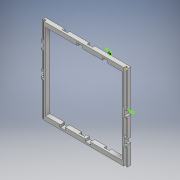
# Autodesk Inventor part: Female_Final
Saved by Autodesk Inventor 2017 (Build 210142000, 142)
## iProperties
Created: 2018-11-26
Part Number: Female_Final
Material: Generic
Document SubType Name: Modeling
Designer: Ralph
Density: 1 g/cm^3
Appearance: Default
Author: Ralph
Autodesk Inventor part; units mm, degrees
ref_plane "YZ Plane" through (0, 0, 0) normal (1, 0, 0) x (0, 1, 0)
ref_plane "XZ Plane" through (0, 0, 0) normal (0, 1, 0) x (-1, 0, 0)
ref_plane "XY Plane" through (0, 0, 0) normal (0, 0, 1) x (1, 0, 0)
sketch "Sketch1" plane through (0, 0, 0) normal (0, 1, 0) x (-1, 0, 0)
  line L0 (0, 0) -> (100, 0)
  line L1 (100, 0) -> (100, -100)
  line L2 (100, -100) -> (0, -100)
  line L3 (0, -100) -> (0, 0)
  line L4 (5, -5) -> (95, -5)
  line L5 (95, -5) -> (95, -95)
  line L6 (95, -95) -> (5, -95)
  line L7 (5, -95) -> (5, -5)
  line L8 (0, 0) -> (0, -5)
  line L9 (0, -5) -> (5, -5)
  dimension "d0" = 100
  dimension "d1" = 100
  dimension "d2" = 90
  dimension "d3" = 90
  dimension "d4" = 5
  dimension "d5" = 5
  constraints: 20 end point, 4 parallel, 3 perpendicular, 2 horizontal, 1 point on line
  measures "d0" distance of L1.end L2.end
  measures "d1" distance of L0.end L1.end
  measures "d2" distance of L5.end L6.end
  measures "d3" distance of L4.end L5.end
  measures "d4" distance between parallel lines of L0 L9
  measures "d5" distance between parallel lines of L3 L7
extrude "Extrusion1" add sketch "Sketch1" along normal blind 5
sketch "Sketch2" plane through (0, 0, 0) normal (0, -1, 0) x (1, 0, 0)
  circle A0 centre (-20, 6) radius 2
  line L0 (-20, 6) -> (-23.9485, 9.8906)
  line L1 (-23.9485, 9.8906) -> (-21.7943, 9.8906)
  line L2 (-21.7943, 9.8906) -> (-23.9485, 9.8906)
  line L3 (-23.9485, 9.8906) -> (-23.9485, 7.9453)
  arc A1 (2.0531, -40.1608) -> (5.7851, -40.1608) centre (3.9191, -39.7302) ccw
  arc A2 (9.4213, -40.1608) -> (5.7851, -40.1608) centre (7.6032, -41.1873) ccw
  point P0 (0, 0)
  dimension "d8" = 4
  constraints: 8 end point, 4 point on circle, 3 centre point, 1 collinear, 1 horizontal, 1 vertical
  measures "d8" diameter of A0
sketch "Sketch3" plane through (0, 0, 0) normal (0, -1, 0) x (1, 0, 0)
  line L0 (0, 0) -> (0, -100) projected
  line L1 (0, 0) -> (0, -5)
  line L2 (0, -5) -> (-20, -5)
  line L3 (-5, -5) -> (-95, -5) projected
  line L4 (-20, -5) -> (-30, -5)
  line L5 (-30, -5) -> (-50, -5)
  line L6 (-50, -5) -> (-60, -5)
  line L7 (-100, -100) -> (-100, 0) projected
  line L8 (-100, -100) -> (-100, -95)
  line L9 (-100, -95) -> (-80, -95)
  line L10 (-95, -95) -> (-5, -95) projected
  line L11 (-80, -95) -> (-70, -95)
  line L12 (-70, -95) -> (-50, -95)
  line L13 (-50, -95) -> (-40, -95)
  line L14 (-20, -5) -> (-22.75, -5)
  line L15 (-22.75, -5) -> (-28.25, -5)
  line L16 (-28.25, -5) -> (-28.25, -2.25)
  line L17 (-28.25, -2.25) -> (-22.75, -2.25)
  line L18 (-22.75, -2.25) -> (-22.75, -5)
  line L19 (-60, -5) -> (-57.25, -5)
  line L20 (-57.25, -5) -> (-51.75, -5)
  line L21 (-51.75, -5) -> (-51.75, -2.25)
  line L22 (-51.75, -2.25) -> (-57.25, -2.25)
  line L23 (-57.25, -2.25) -> (-57.25, -5)
  line L24 (-40, -95) -> (-42.75, -95)
  line L25 (-42.75, -95) -> (-48.25, -95)
  line L26 (-48.25, -95) -> (-48.25, -97.75)
  line L27 (-48.25, -97.75) -> (-42.75, -97.75)
  line L28 (-42.75, -97.75) -> (-42.75, -95)
  line L29 (-80, -95) -> (-77.25, -95)
  line L30 (-77.25, -95) -> (-71.75, -95)
  line L31 (-71.75, -95) -> (-71.75, -97.75)
  line L32 (-71.75, -97.75) -> (-77.25, -97.75)
  line L33 (-77.25, -97.75) -> (-77.25, -95)
  dimension "d9" = 5
  dimension "d10" = 20
  dimension "d11" = 10
  dimension "d12" = 20
  dimension "d13" = 10
  dimension "d14" = 5
  dimension "d15" = 20
  dimension "d16" = 10
  dimension "d17" = 20
  dimension "d18" = 10
  dimension "d19" = 2.75
  dimension "d20" = 5.5
  dimension "d21" = 2.75
  dimension "d22" = 2.75
  dimension "d23" = 5.5
  dimension "d24" = 2.75
  dimension "d25" = 2.75
  dimension "d26" = 5.5
  dimension "d27" = 2.75
  dimension "d28" = 2.75
  dimension "d29" = 5.5
  dimension "d30" = 2.75
  constraints: 60 end point, 13 point on line, 8 parallel, 4 horizontal, 4 perpendicular, 1 midpoint
  measures "d9" distance of L0.start L1.end
  measures "d10" distance of L1.end L2.end
  measures "d11" distance of L2.end L4.end
  measures "d12" distance of L4.end L5.end
  measures "d13" distance of L5.end L6.end
  measures "d14" distance of L7.start L8.end
  measures "d15" distance of L8.end L9.end
  measures "d16" distance of L9.end L11.end
  measures "d17" distance of L11.end L12.end
  measures "d18" distance of L12.end L13.end
  measures "d19" distance of L2.end L14.end
  measures "d20" distance of L16.end L17.end
  measures "d21" distance of L15.end L16.end
  measures "d22" distance of L6.end L19.end
  measures "d23" distance of L22.end L21.end
  measures "d24" distance of L21.end L20.end
  measures "d25" distance of L13.end L24.end
  measures "d26" distance of L27.end L26.end
  measures "d27" distance of L26.end L25.end
  measures "d28" distance of L9.end L29.end
  measures "d29" distance of L31.end L32.end
  measures "d30" distance of L30.end L31.end
extrude "Extrusion2" cut sketch "Sketch3" against normal blind 3
sketch "Sketch4" plane through (0, 0, 0) normal (0, -1, 0) x (1, 0, 0)
  line L0 (0, 0) -> (-3.25, 0)
  line L1 (-3.25, 0) -> (-3.25, -100)
  line L2 (-3.25, -100) -> (0, -100)
  line L3 (0, -100) -> (0, 0)
  line L4 (-100, 0) -> (0, 0) projected
  line L5 (-100, 0) -> (-96.75, 0)
  line L6 (-96.75, 0) -> (-96.75, -100)
  line L7 (-96.75, -100) -> (-100, -100)
  line L8 (-100, -100) -> (-100, 0)
  dimension "d33" = 3.25
  dimension "d34" = 100
  dimension "d35" = 3.25
  dimension "d36" = 100
  constraints: 16 end point, 4 parallel, 2 horizontal, 2 perpendicular
  measures "d33" distance of L2.end L1.end
  measures "d34" distance of L1.end L0.end
  measures "d35" distance of L6.end L7.end
  measures "d36" distance of L5.end L6.end
extrude "Extrusion3" cut sketch "Sketch4" against normal blind 1
sketch "Sketch5" plane through (0, 1, 0) normal (0, -1, 0) x (1, 0, 0)
  line L0 (-3.25, -100) -> (-3.25, 0) projected
  line L1 (-3.25, 0) -> (-1.25, 0)
  line L2 (-1.25, 0) -> (-1.25, -100)
  line L3 (-1.25, -100) -> (-3.25, -100)
  line L4 (-3.25, -100) -> (-3.25, 0)
  line L5 (-96.75, 0) -> (-3.25, 0) projected
  line L6 (-96.75, 0) -> (-98.75, 0)
  line L7 (-98.75, 0) -> (-98.75, -100)
  line L8 (-98.75, -100) -> (-96.75, -100)
  line L9 (-96.75, -100) -> (-96.75, 0)
  point P0 (0, 0)
  dimension "d39" = 2
  dimension "d40" = 100
  dimension "d41" = 2
  dimension "d42" = 100
  constraints: 16 end point, 4 parallel, 2 horizontal, 2 perpendicular
  measures "d39" distance of L2.end L3.end
  measures "d40" distance of L1.end L2.end
  measures "d41" distance of L8.end L7.end
  measures "d42" distance of L7.end L6.end
extrude "Extrusion4" cut sketch "Sketch5" against normal blind 1.75
sketch "Sketch6" plane through (-5, 5, -5) normal (0, 0, -1) x (-1, 0, 0)
  line L0 (17.75, -2) -> (23.25, -2) projected
  line L1 (23.25, -2) -> (17.25, -2)
  line L2 (17.25, -2) -> (17.25, 0)
  line L3 (17.25, 0) -> (23.25, 0)
  line L4 (23.25, 0) -> (23.25, -2)
  line L5 (46.75, -5) -> (46.75, -2) projected
  line L6 (46.75, -2) -> (52.75, -2)
  line L7 (52.75, -2) -> (52.75, 0)
  line L8 (52.75, 0) -> (46.75, 0)
  line L9 (46.75, 0) -> (46.75, -2)
  point P0 (-5, -5)
  dimension "d47" = 6
  dimension "d48" = 2
  dimension "d49" = 6
  dimension "d50" = 2
  constraints: 16 end point, 4 parallel, 2 horizontal, 2 perpendicular
  measures "d47" distance of L2.end L3.end
  measures "d48" distance of L1.end L2.end
  measures "d49" distance of L8.end L7.end
  measures "d50" distance of L7.end L6.end
extrude "Extrusion5" cut sketch "Sketch6" against normal blind 2.75
sketch "Sketch7" plane through (-95, 5, -95) normal (0, 0, 1) x (1, 0, 0)
  line L0 (17.75, -2) -> (23.25, -2) projected
  line L1 (23.25, -2) -> (17.25, -2)
  line L2 (17.25, -2) -> (17.25, 0)
  line L3 (17.25, 0) -> (23.25, 0)
  line L4 (23.25, 0) -> (23.25, -2)
  line L5 (46.75, -5) -> (46.75, -2) projected
  line L6 (46.75, -2) -> (52.75, -2)
  line L7 (52.75, -2) -> (52.75, 0)
  line L8 (52.75, 0) -> (46.75, 0)
  line L9 (46.75, 0) -> (46.75, -2)
  point P0 (95, -5)
  dimension "d53" = 6
  dimension "d54" = 2
  dimension "d55" = 6
  dimension "d56" = 2
  constraints: 16 end point, 4 parallel, 2 horizontal, 2 perpendicular
  measures "d53" distance of L2.end L3.end
  measures "d54" distance of L1.end L2.end
  measures "d55" distance of L8.end L7.end
  measures "d56" distance of L7.end L6.end
extrude "Extrusion6" cut sketch "Sketch7" against normal blind 2.75
fillet "Fillet1" radius 1 4 edges at (-77.25, 0, -96.375) (-42.75, 0, -96.375) (-22.75, 0, -3.625) (-57.25, 0, -3.625)
sketch "Sketch8" plane through (-100, 5, 0) normal (0, 0, 1) x (1, 0, 0)
  line L0 (0, -4) -> (0, 0) projected
  line L1 (0, 0) -> (20, 0)
  line L2 (20, 0) -> (30, 0)
  line L3 (30, 0) -> (50, 0)
  line L4 (50, 0) -> (60, 0)
  line L5 (60, 0) -> (57, 0)
  line L6 (0, 0) -> (100, 0) projected
  line L7 (57, 0) -> (51.5, 0)
  line L8 (51.5, 0) -> (51.5, -2.75)
  line L9 (51.5, -2.75) -> (57, -2.75)
  line L10 (57, -2.75) -> (57, 0)
  line L11 (20, 0) -> (23, 0)
  line L12 (23, 0) -> (28.5, 0)
  line L13 (28.5, 0) -> (28.5, -2.75)
  line L14 (28.5, -2.75) -> (23, -2.75)
  line L15 (23, -2.75) -> (23, 0)
  point P0 (100, -5)
  dimension "d60" = 20
  dimension "d61" = 10
  dimension "d62" = 20
  dimension "d63" = 10
  dimension "d64" = 3
  dimension "d65" = 5.5
  dimension "d66" = 2.75
  dimension "d67" = 3
  dimension "d68" = 5.5
  dimension "d69" = 2.75
  constraints: 28 end point, 5 point on line, 4 parallel, 3 horizontal, 2 perpendicular
  measures "d60" distance of L0.end L1.end
  measures "d61" distance of L1.end L2.end
  measures "d62" distance of L2.end L3.end
  measures "d63" distance of L3.end L4.end
  measures "d64" distance of L4.end L5.end
  measures "d65" distance of L9.end L8.end
  measures "d66" distance of L8.end L7.end
  measures "d67" distance of L1.end L11.end
  measures "d68" distance of L13.end L14.end
  measures "d69" distance of L12.end L13.end
extrude "Extrusion7" cut sketch "Sketch8" against normal blind 3
sketch "Sketch9" plane through (0, 5, 0) normal (0, 1, 0) x (1, 0, 0)
  line L0 (-43, 3) -> (-48.5, 3) projected
  line L1 (-48.5, 3) -> (-42.5, 3)
  line L2 (-42.5, 3) -> (-42.5, 5)
  line L3 (-42.5, 5) -> (-48.5, 5)
  line L4 (-48.5, 5) -> (-48.5, 3)
  line L5 (-71.5, 3) -> (-77.5, 3)
  line L6 (-77.5, 3) -> (-77.5, 5)
  line L7 (-77.5, 5) -> (-71.5, 5)
  line L8 (-71.5, 5) -> (-71.5, 3)
  point P0 (0, 0)
  dimension "d72" = 6
  dimension "d73" = 2
  dimension "d74" = 6
  dimension "d75" = 2
  constraints: 16 end point, 4 parallel, 2 horizontal, 2 perpendicular
  measures "d72" distance of L3.end L2.end
  measures "d73" distance of L2.end L1.end
  measures "d74" distance of L6.end L7.end
  measures "d75" distance of L5.end L6.end
extrude "Extrusion8" cut sketch "Sketch9" against normal blind 2.75
sketch "Sketch10" plane through (0, 5, -100) normal (0, 0, -1) x (-1, 0, 0)
  line L0 (0, 0) -> (100, 0) projected
  line L1 (0, 0) -> (20, 0)
  line L2 (20, 0) -> (30, 0)
  line L3 (30, 0) -> (50, 0)
  line L4 (50, 0) -> (60, 0)
  line L5 (60, 0) -> (57, 0)
  line L6 (57, 0) -> (51.5, 0)
  line L7 (51.5, 0) -> (51.5, -2.75)
  line L8 (51.5, -2.75) -> (57, -2.75)
  line L9 (57, -2.75) -> (57, 0)
  line L10 (20, 0) -> (23, 0)
  line L11 (23, 0) -> (28.5, 0)
  line L12 (28.5, 0) -> (28.5, -2.75)
  line L13 (28.5, -2.75) -> (23, -2.75)
  line L14 (23, -2.75) -> (23, 0)
  point P0 (0, -5)
  dimension "d78" = 20
  dimension "d79" = 10
  dimension "d80" = 20
  dimension "d81" = 10
  dimension "d82" = 3
  dimension "d83" = 5.5
  dimension "d84" = 2.75
  dimension "d85" = 3
  dimension "d86" = 5.5
  dimension "d87" = 2.75
  constraints: 28 end point, 5 point on line, 4 parallel, 2 horizontal, 2 perpendicular, 1 midpoint
  measures "d78" distance of L0.start L1.end
  measures "d79" distance of L1.end L2.end
  measures "d80" distance of L2.end L3.end
  measures "d81" distance of L3.end L4.end
  measures "d82" distance of L4.end L5.end
  measures "d83" distance of L8.end L7.end
  measures "d84" distance of L7.end L6.end
  measures "d85" distance of L1.end L10.end
  measures "d86" distance of L12.end L13.end
  measures "d87" distance of L11.end L12.end
extrude "Extrusion9" cut sketch "Sketch10" against normal blind 3
sketch "Sketch11" plane through (0, 5, 0) normal (0, 1, 0) x (1, 0, 0)
  line L0 (-51.5, 97) -> (-57, 97) projected
  line L1 (-51.5, 97) -> (-57.5, 97)
  line L2 (-57.5, 97) -> (-57.5, 95)
  line L3 (-57.5, 95) -> (-51.5, 95)
  line L4 (-51.5, 95) -> (-51.5, 97)
  line L5 (-23, 97) -> (-28.5, 97) projected
  line L6 (-28.5, 97) -> (-22.5, 97)
  line L7 (-22.5, 97) -> (-22.5, 95)
  line L8 (-22.5, 95) -> (-28.5, 95)
  line L9 (-28.5, 95) -> (-28.5, 97)
  point P0 (0, 0)
  dimension "d90" = 6
  dimension "d91" = 2
  dimension "d92" = 6
  dimension "d93" = 2
  constraints: 16 end point, 4 parallel, 2 horizontal, 2 perpendicular
  measures "d90" distance of L3.end L2.end
  measures "d91" distance of L2.end L1.end
  measures "d92" distance of L7.end L8.end
  measures "d93" distance of L6.end L7.end
extrude "Extrusion10" cut sketch "Sketch11" against normal blind 2.75
fillet "Fillet2" radius 1 4 edges at (-57, 3.625, -100) (-23, 3.625, -100) (-77, 3.625, 0) (-43, 3.625, 0)
sketch "Sketch12" plane through (0, 2.75, 0) normal (0, -1, 0) x (1, 0, 0)
  line L0 (-1.25, -100) -> (-3.25, -100) projected
  line L1 (-1.25, -100) -> (-1.25, -80)
  line L2 (-1.25, 0) -> (-1.25, -100) projected
  line L3 (-1.25, -80) -> (-1.25, -70)
  line L4 (-1.25, -70) -> (-1.25, -50)
  line L5 (-1.25, -50) -> (-1.25, -40)
  line L6 (-3.25, -100) -> (-3.25, 0) projected
  line L7 (-1.25, -40) -> (-3.25, -40)
  line L8 (-3.25, -40) -> (-3.25, -50)
  line L9 (-3.25, -50) -> (-1.25, -50)
  line L10 (-1.25, -50) -> (-1.25, -40)
  line L11 (-1.25, -70) -> (-3.25, -70)
  line L12 (-3.25, -70) -> (-3.25, -80)
  line L13 (-3.25, -80) -> (-1.25, -80)
  line L14 (-1.25, -80) -> (-1.25, -70)
  line L15 (-98.75, -100) -> (-98.75, 0) projected
  line L16 (-98.75, 0) -> (-98.75, -20)
  line L17 (-98.75, -20) -> (-98.75, -30)
  line L18 (-98.75, -30) -> (-98.75, -50)
  line L19 (-98.75, -50) -> (-98.75, -60)
  line L20 (-96.75, 0) -> (-96.75, -100) projected
  line L21 (-98.75, -60) -> (-96.75, -60)
  line L22 (-96.75, -60) -> (-96.75, -50)
  line L23 (-96.75, -50) -> (-98.75, -50)
  line L24 (-98.75, -50) -> (-98.75, -60)
  line L25 (-98.75, -20) -> (-96.75, -20)
  line L26 (-96.75, -20) -> (-96.75, -30)
  line L27 (-96.75, -30) -> (-98.75, -30)
  line L28 (-98.75, -30) -> (-98.75, -20)
  point P0 (0, 0)
  dimension "d97" = 20
  dimension "d98" = 10
  dimension "d99" = 20
  dimension "d100" = 10
  dimension "d103" = 20
  dimension "d104" = 10
  dimension "d105" = 20
  dimension "d106" = 10
  constraints: 48 end point, 10 point on line, 8 parallel, 4 horizontal, 4 perpendicular, 2 midpoint
  measures "d97" distance of L0.start L1.end
  measures "d98" distance of L1.end L3.end
  measures "d99" distance of L3.end L4.end
  measures "d100" distance of L4.end L5.end
  measures "d103" distance of L15.end L16.end
  measures "d104" distance of L16.end L17.end
  measures "d105" distance of L17.end L18.end
  measures "d106" distance of L18.end L19.end
extrude "Extrusion11" add sketch "Sketch12" along normal blind 2.75 contours L13 L6 L11 L2 | L9 L6 L7 L2 | L15 L23 L20 L21 | L15 L25 L20 L27
sketch "Sketch13" plane through (-98.75, 0, -60) normal (-1, 0, 0) x (0, 0, 1)
  line L0 (60, 0) -> (40, 0) projected
  line L1 (40, 0) -> (30, 0)
  line L2 (30, 0) -> (30, 1)
  line L3 (30, 1) -> (40, 1)
  line L4 (40, 1) -> (40, 0)
  line L5 (30, 0) -> (10, 0) projected
  line L6 (10, 0) -> (0, 0)
  line L7 (0, 0) -> (0, 1)
  line L8 (0, 1) -> (10, 1)
  line L9 (10, 1) -> (10, 0)
  dimension "d107" = 10
  dimension "d108" = 1
  dimension "d109" = 10
  dimension "d110" = 1
  constraints: 16 end point, 4 parallel, 2 horizontal, 2 perpendicular
  measures "d107" distance of L2.end L3.end
  measures "d108" distance of L1.end L2.end
  measures "d109" distance of L7.end L8.end
  measures "d110" distance of L6.end L7.end
extrude "Extrusion12" add sketch "Sketch13" along normal blind 1.25
sketch "Sketch14" plane through (-1.25, 0, -70) normal (1, 0, 0) x (0, 0, -1)
  line L0 (-65, 0) -> (25, 0) projected
  line L1 (-20, 0) -> (-30, 0)
  line L2 (-30, 0) -> (-30, 1)
  line L3 (-30, 1) -> (-20, 1)
  line L4 (-20, 1) -> (-20, 0)
  line L5 (0, 0) -> (10, 0)
  line L6 (10, 0) -> (10, 1)
  line L7 (10, 1) -> (0, 1)
  line L8 (0, 1) -> (0, 0)
  point P0 (-70, 0)
  dimension "d113" = 10
  dimension "d114" = 1
  dimension "d115" = 10
  dimension "d116" = 1
  constraints: 16 end point, 4 parallel, 2 horizontal, 2 perpendicular, 1 midpoint
  measures "d113" distance of L2.end L3.end
  measures "d114" distance of L1.end L2.end
  measures "d115" distance of L7.end L6.end
  measures "d116" distance of L6.end L5.end
extrude "Extrusion13" add sketch "Sketch14" along normal blind 1.25
sketch "Sketch15" plane through (0, 5, 0) normal (0, 1, 0) x (1, 0, 0)
  line L0 (0, 0) -> (0, 100) projected
  line L1 (0, 100) -> (0, 80)
  line L2 (0, 80) -> (0, 70)
  line L3 (0, 70) -> (0, 50)
  line L4 (0, 50) -> (0, 40)
  line L5 (0, 40) -> (0, 43)
  line L6 (0, 40) -> (0, 50) projected
  line L7 (0, 43) -> (-2.75, 43)
  line L8 (-2.75, 43) -> (-2.75, 48.5)
  line L9 (-2.75, 48.5) -> (0, 48.5)
  line L10 (0, 48.5) -> (0, 43)
  line L11 (0, 80) -> (0, 77)
  line L12 (0, 70) -> (0, 80) projected
  line L13 (0, 77) -> (-2.75, 77)
  line L14 (-2.75, 77) -> (-2.75, 71.5)
  line L15 (-2.75, 71.5) -> (0, 71.5)
  line L16 (0, 71.5) -> (0, 77)
  line L17 (-100, 20) -> (-100, 0) projected
  line L18 (-100, 0) -> (-100, 20)
  line L19 (-100, 30) -> (-100, 20) projected
  line L20 (-100, 20) -> (-100, 30)
  line L21 (-100, 50) -> (-100, 30) projected
  line L22 (-100, 30) -> (-100, 50)
  line L23 (-100, 60) -> (-100, 50) projected
  line L24 (-100, 50) -> (-100, 60)
  line L25 (-96.75, 60) -> (-100, 60) projected
  line L26 (-100, 60) -> (-100, 57)
  line L27 (-100, 57) -> (-97.25, 57)
  line L28 (-97.25, 57) -> (-97.25, 51.5)
  line L29 (-97.25, 51.5) -> (-100, 51.5)
  line L30 (-100, 51.5) -> (-100, 57)
  line L31 (-96.75, 20) -> (-100, 20) projected
  line L32 (-100, 20) -> (-100, 23)
  line L33 (-100, 23) -> (-97.25, 23)
  line L34 (-97.25, 23) -> (-97.25, 28.5)
  line L35 (-97.25, 28.5) -> (-100, 28.5)
  line L36 (-100, 28.5) -> (-100, 23)
  dimension "d119" = 20
  dimension "d120" = 10
  dimension "d121" = 20
  dimension "d122" = 10
  dimension "d123" = 3
  dimension "d124" = 2.75
  dimension "d125" = 5.5
  dimension "d126" = 3
  dimension "d127" = 2.75
  dimension "d128" = 5.5
  dimension "d129" = 20
  dimension "d130" = 10
  dimension "d131" = 20
  dimension "d132" = 10
  dimension "d133" = 3
  dimension "d134" = 2.75
  dimension "d135" = 5.5
  dimension "d136" = 3
  dimension "d137" = 2.75
  dimension "d138" = 5.5
  constraints: 56 end point, 8 parallel, 7 point on line, 4 collinear, 4 horizontal, 4 perpendicular, 1 midpoint
  measures "d119" distance of L0.end L1.end
  measures "d120" distance of L1.end L2.end
  measures "d121" distance of L2.end L3.end
  measures "d122" distance of L3.end L4.end
  measures "d123" distance of L4.end L5.end
  measures "d124" distance of L8.end L9.end
  measures "d125" distance of L7.end L8.end
  measures "d126" distance of L1.end L11.end
  measures "d127" distance of L15.end L14.end
  measures "d128" distance of L14.end L13.end
  measures "d129" distance of L17.end L17.start
  measures "d130" distance of L17.start L19.start
  measures "d131" distance of L19.start L21.start
  measures "d132" distance of L21.start L23.start
  measures "d133" distance of L23.start L26.end
  measures "d134" distance of L28.end L29.end
  measures "d135" distance of L27.end L28.end
  measures "d136" distance of L17.start L32.end
  measures "d137" distance of L35.end L34.end
  measures "d138" distance of L34.end L33.end
extrude "Extrusion14" cut sketch "Sketch15" against normal blind 3
sketch "Sketch16" plane through (0, 1, 0) normal (1, 0, 0) x (0, 0, -1)
  line L0 (43, 1) -> (48.5, 1) projected
  line L1 (48.5, 1) -> (42.5, 1)
  line L2 (42.5, 1) -> (42.5, -1)
  line L3 (42.5, -1) -> (48.5, -1)
  line L4 (48.5, -1) -> (48.5, 1)
  line L5 (71.5, 4) -> (71.5, 1) projected
  line L6 (71.5, 1) -> (77.5, 1)
  line L7 (77.5, 1) -> (77.5, -1)
  line L8 (77.5, -1) -> (71.5, -1)
  line L9 (71.5, -1) -> (71.5, 1)
  point P0 (0, -1)
  dimension "d141" = 6
  dimension "d142" = 2
  dimension "d143" = 6
  dimension "d144" = 2
  constraints: 16 end point, 4 parallel, 2 horizontal, 2 perpendicular
  measures "d141" distance of L3.end L2.end
  measures "d142" distance of L2.end L1.end
  measures "d143" distance of L7.end L8.end
  measures "d144" distance of L6.end L7.end
extrude "Extrusion15" cut sketch "Sketch16" against normal blind 2.75
sketch "Sketch17" plane through (-100, 1, -100) normal (-1, 0, 0) x (0, 0, 1)
  line L0 (71.5, 1) -> (71.5, 4) projected
  line L1 (71.5, 1) -> (77.5, 1)
  line L2 (77.5, 1) -> (77.5, -1)
  line L3 (77.5, -1) -> (71.5, -1)
  line L4 (71.5, -1) -> (71.5, 1)
  line L5 (48.5, 4) -> (48.5, 1) projected
  line L6 (48.5, 1) -> (42.5, 1)
  line L7 (42.5, 1) -> (42.5, -1)
  line L8 (42.5, -1) -> (48.5, -1)
  line L9 (48.5, -1) -> (48.5, 1)
  point P0 (100, -1)
  dimension "d147" = 6
  dimension "d148" = 2
  dimension "d149" = 6
  dimension "d150" = 2
  constraints: 16 end point, 4 parallel, 2 horizontal, 2 perpendicular
  measures "d147" distance of L2.end L3.end
  measures "d148" distance of L1.end L2.end
  measures "d149" distance of L8.end L7.end
  measures "d150" distance of L7.end L6.end
extrude "Extrusion16" cut sketch "Sketch17" against normal blind 2.75
body "Solid1"
